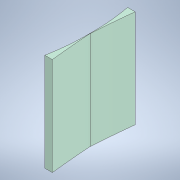
# Autodesk Inventor part: rendering_light_sheet
Saved by Autodesk Inventor 2021 (Build 250183000, 183)
## iProperties
Created: 2021-06-18
Part Number: rendering_light_sheet
Material: Generic
Document SubType Name: Modeling
Designer: MicroscopyInnovation
Density: 1 g/cm^3
Appearance: Default
Author: MicroscopyInnovation
Autodesk Inventor part; units mm, degrees
ref_plane "YZ Plane" through (0, 0, 0) normal (1, 0, 0) x (0, 1, 0)
ref_plane "XZ Plane" through (0, 0, 0) normal (0, 1, 0) x (-1, 0, 0)
ref_plane "XY Plane" through (0, 0, 0) normal (0, 0, 1) x (1, 0, 0)
sketch "Sketch1" plane through (0, 0, 0) normal (0, 1, 0) x (-1, 0, 0)
  arc A0 (7.6582, 84.6765) -> (0.25, 0) centre (430.2204, 5.0448) ccw
  line L0 (0.25, 0) -> (7.6582, 84.6765) construction
  line L1 (0.25, 0) -> (85.25, 0) construction
  arc A1 (0.25, 0) -> (7.6582, -84.6765) centre (430.2204, -5.0448) ccw
  line L2 (0.25, 0) -> (7.6582, -84.6765) construction
  line L3 (0.25, 0) -> (85.25, 0) construction
  arc A2 (-0.25, 0) -> (-7.6582, 84.6765) centre (-1809.956, -115.6664) ccw
  line L4 (-0.25, 0) -> (-7.6582, 84.6765) construction
  line L5 (-0.25, 0) -> (84.75, 0) construction
  line L6 (-0.25, 0) -> (84.75, 0) construction
  arc A3 (-7.6582, -84.6765) -> (-0.25, 0) centre (-1823.7815, 116.876) ccw
  line L7 (-0.25, 0) -> (-7.6582, -84.6765) construction
  line L8 (-0.25, 0) -> (84.75, 0) construction
  line L9 (7.6582, 84.6765) -> (-7.6582, 84.6765)
  line L10 (7.6582, -84.6765) -> (-7.6582, -84.6765)
  point P0 (0, 0)
  dimension "d0" = 85
  dimension "d1" = 85
  dimension "d2" = 430
  dimension "d3" = 85
  dimension "d4" = 85
  dimension "d5" = 430
  dimension "d6" = 85
  dimension "d7" = 95
  dimension "d10" = 85
  dimension "d11" = 95
  constraints: 22 end point, 8 point on circle, 6 horizontal, 4 centre point, 4 equal length, 1 tangent
  measures "d0" distance of L0.start L0.end
  measures "d1" angle of L1 L0
  measures "d2" radius of A0
  measures "d3" distance of L0.start L2.end
  measures "d4" angle of L2 L3
  measures "d5" radius of A1
  measures "d6" distance of L4.start L4.end
  measures "d7" angle of L5 L4
  measures "d10" distance of L4.start L7.end
  measures "d11" angle of L7 L8
extrude "Extrusion1" add sketch "Sketch1" along normal blind 200
body "Solid1"
